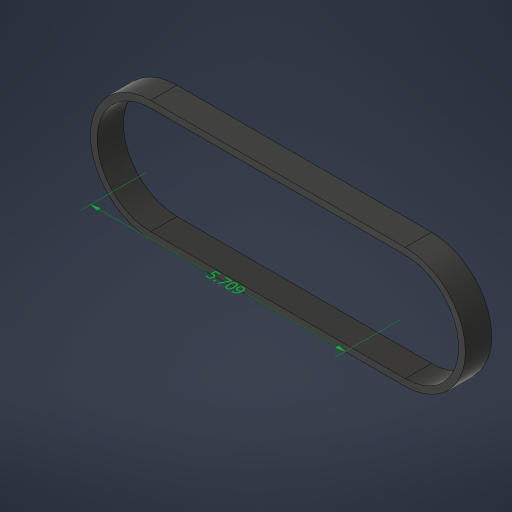
# Autodesk Inventor part: Belt Calculator
Saved by Autodesk Inventor 2023.1 (Build 271208000, 208)
## iProperties
Created: 2021-02-26
Part Number: Belt Calculator
Material: Nylon 6/6
Document SubType Name: Modeling
Designer: Byron Robotics
Density: 1.13 g/cm^3
Appearance: Smooth - Black
Mass: 31.7882 g
Surface Area: 185.567 cm^2
Volume: 28.1311 cm^3
Description: HTD Belt Calculator
DocNumber: Belt Calculator.ipt
Folder: .
VDS_Category: CAD
Author: Byron Robotics
Revision Number: D
Autodesk Inventor part; units mm, degrees
ref_plane "YZ Plane" through (0, 0, 0) normal (1, 0, 0) x (0, 1, 0)
ref_plane "XZ Plane" through (0, 0, 0) normal (0, 1, 0) x (-1, 0, 0)
ref_plane "XY Plane" through (0, 0, 0) normal (0, 0, 1) x (1, 0, 0)
sketch "BeltOuterProfile" plane through (0, 0, 0) normal (0, 0, 1) x (1, 0, 0)
  arc A0 (0, 34.2925) -> (0, -34.2925) centre (0, 0) ccw
  arc A1 (145, -34.2925) -> (145, 34.2925) centre (145, 0) ccw
  line L0 (0, 34.2925) -> (145, 34.2925)
  line L1 (0, -34.2925) -> (145, -34.2925)
  line L2 (0, 0) -> (500, 0) construction
  line L3 (145, 34.2925) -> (145, 0) construction
  line L4 (145, 0) -> (145, -34.2925) construction
  line L5 (0, 0) -> (0, 34.2925) construction
  line L6 (0, 0) -> (0, -34.2925) construction
  dimension "BeltLength" = 500
  dimension "CenterDistance" = 145
  dimension "d24" = 34.2925
  dimension "d25" = 34.2925
  constraints: 14 end point, 5 point on circle, 4 tangent, 2 centre point, 1 coincident, 1 horizontal, 1 horizontal alignment
  measures "BeltLength" distance of L2.start L2.end
  measures "CenterDistance" distance of L3.end point (0, 0)
  measures "d24" radius of A0
  measures "d25" radius of A1
extrude "BeltWidth" add sketch "BeltOuterProfile" along normal blind 15
sketch "BeltThickness" plane through (0, 0, 15) normal (0, 0, 1) x (1, 0, 0)
  arc A0 (0, 34.2925) -> (0, -34.2925) centre (0, 0) ccw projected
  line L0 (0, -34.2925) -> (145, -34.2925) projected
  arc A1 (145, -34.2925) -> (145, 34.2925) centre (145, 0) ccw projected
  line L1 (145, 34.2925) -> (0, 34.2925) projected
  arc A2 (0, 30.4925) -> (0, -30.4925) centre (0, 0) ccw
  line L2 (0, -30.4925) -> (145, -30.4925)
  arc A3 (145, -30.4925) -> (145, 30.4925) centre (145, 0) ccw
  line L3 (145, 30.4925) -> (0, 30.4925)
  dimension "d17" = 3.8
  constraints: 4 end point, 4 point on circle, 2 centre point, 3 other
  measures "d17" distance between parallel lines of L1 L3
extrude "BeltInternalAreaCut" cut sketch "BeltThickness" against normal through all contours L3 A3 L2 A2
equation "\"Pulley1WrapLength\" = 1"
equation "\"Pulley2WrapLength\" = 1"
body "Solid2"
